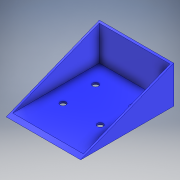
# Autodesk Inventor part: Bucket
Saved by Autodesk Inventor 2020 (Build 240168000, 168)
## iProperties
Created: 2019-10-01
Part Number: Bucket
Material: Aluminum 6061
Document SubType Name: Modeling
Designer: Matt
Mass: 157.818 g
Surface Area: 476.751 cm^2
Volume: 58.451 cm^3
Density: 2.7 g/cm^3
Appearance: Blue - Wall Paint - Glossy
Author: Matt
Autodesk Inventor part; units mm, degrees
ref_plane "YZ Plane" through (0, 0, 0) normal (1, 0, 0) x (0, 1, 0)
ref_plane "XZ Plane" through (0, 0, 0) normal (0, 1, 0) x (-1, 0, 0)
ref_plane "XY Plane" through (0, 0, 0) normal (0, 0, 1) x (1, 0, 0)
sketch "Sketch1" plane through (0, 0, 0) normal (1, 0, 0) x (0, 1, 0)
  line L0 (0, 0) -> (0, -127)
  line L1 (0, -127) -> (50.8, -127)
  line L2 (0, 0) -> (50.8, -127)
  dimension "d0" = 127
  dimension "d1" = 50.8
  constraints: 6 end point, 1 perpendicular, 1 vertical
  measures "d0" distance of L0.start L0.end
  measures "d1" distance of L0.end L1.end
extrude "Extrusion1" add sketch "Sketch1" along normal blind 101.6
shell "Shell1" thickness 2.54 removed faces 1 at (33.8667, 33.8667, -84.6667)
sketch "Sketch2" plane through (0, 0, -127) normal (0, -1, 0) x (1, 0, 0)
  line L0 (0, 127) -> (0, 0) projected
  line L1 (0, 0) -> (101.6, 0) projected
  line L2 (101.6, 127) -> (101.6, 0) projected
  line L3 (0, 127) -> (101.6, 127) projected
  point P0 (25.4, 30.48)
  point P1 (25.4, 74.93)
  point P2 (76.2, 74.93)
  point P3 (76.2, 30.48)
  dimension "d5" = 30.48
  dimension "d6" = 30.48
  dimension "d7" = 25.4
  dimension "d8" = 25.4
  dimension "d9" = 25.4
  dimension "d10" = 25.4
  dimension "d11" = 44.45
  dimension "d12" = 44.45
  measures "d5" distance from line of L1 point (25.4, 30.48)
  measures "d6" distance from line of L1 point (76.2, 30.48)
  measures "d7" distance from line of L2 point (76.2, 74.93)
  measures "d8" distance from line of L0 point (25.4, 74.93)
  measures "d9" distance from line of L0 point (25.4, 30.48)
  measures "d10" distance from line of L2 point (76.2, 30.48)
  measures "d11" distance of point (25.4, 74.93) point (25.4, 30.48)
  measures "d12" distance of point (76.2, 30.48) point (76.2, 74.93)
hole "Hole1" at (25.4, 0, -96.52) at (25.4, 0, -52.07) at (76.2, 0, -52.07) at (76.2, 0, -96.52) direction (0, 1, 0) diameter 8 depth 19.05 tip angle 118
equation "\"d6\" = d5"
equation "\"d8\" = d7"
equation "\"d9\" = d7"
equation "\"d10\" = d7"
equation "\"d12\" = d11"
body "Solid1"
